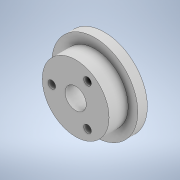
# Autodesk Inventor part: Tractor_Static
Saved by Autodesk Inventor 2022 (Build 260153070, 153G)
## iProperties
Created: 2022-03-05
Part Number: Tractor_Static
Material: Generic
Document SubType Name: Modeling
Designer: a laptop
Density: 1 g/cm^3
Appearance: Default
Author: a laptop
Autodesk Inventor part; units mm, degrees
ref_plane "YZ Plane" through (0, 0, 0) normal (1, 0, 0) x (0, 1, 0)
ref_plane "XZ Plane" through (0, 0, 0) normal (0, 1, 0) x (-1, 0, 0)
ref_plane "XY Plane" through (0, 0, 0) normal (0, 0, 1) x (1, 0, 0)
sketch "Sketch1" plane through (0, 0, 0) normal (0, 0, 1) x (1, 0, 0)
  circle A0 centre (0, 0) radius 45
  circle A1 centre (0, 0) radius 34.925
  circle A2 centre (0, 0) radius 11.075
  dimension "d0" = 90
  dimension "d1" = 69.85
  dimension "d2" = 22.15
  constraints: 3 centre point, 3 coincident
  measures "d0" diameter of A0
  measures "d1" diameter of A1
  measures "d2" diameter of A2
extrude "Extrusion1" add sketch "Sketch1" along normal blind 20 contours A1
extrude "Extrusion2" add sketch "Sketch1" against normal blind 10 contours A0
sketch "Sketch2" plane through (0, 0, 20) normal (0, 0, 1) x (1, 0, 0)
  circle A0 centre (12.4625, 21.5857) radius 4
  circle A1 centre (-24.925, 0) radius 4
  circle A2 centre (12.4625, -21.5857) radius 4
  line L0 (-24.925, 0) -> (12.4625, 21.5857) construction
  line L1 (12.4625, 21.5857) -> (12.4625, -21.5857) construction
  line L2 (12.4625, -21.5857) -> (-24.925, 0) construction
  line L3 (12.4625, 21.5857) -> (17.4625, 30.2459) construction
  circle A3 centre (0, 0) radius 34.925 projected
  line L4 (-24.925, 0) -> (-34.925, 0) construction
  line L5 (12.4625, -21.5857) -> (17.4625, -30.2459) construction
  dimension "d7" = 8
  dimension "d8" = 10
  constraints: 12 end point, 4 equal length, 3 centre point, 3 line through centre, 3 point on circle, 2 equal radius, 1 horizontal
  measures "d7" diameter of A0
  measures "d8" distance of L0.end L3.end
extrude "Extrusion3" cut sketch "Sketch2" against normal blind 15 contours A0 | A1 | A2
body "Solid1"
